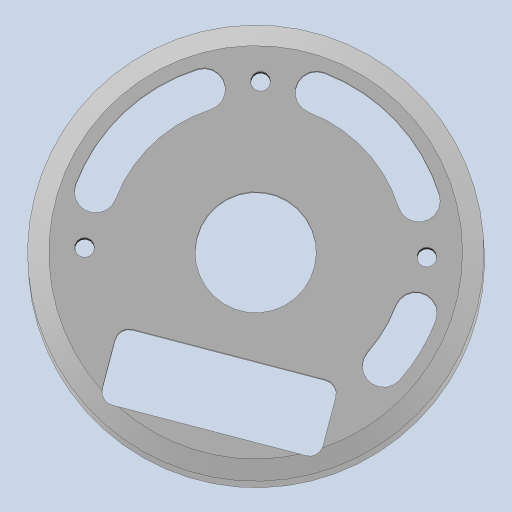
# Autodesk Inventor part: PotCover-Shorter
Saved by Autodesk Inventor 2023 (Build 270158000, 158)
## iProperties
Created: 2024-02-10
Part Number: PotCover-Shorter
Material: Generic
Document SubType Name: Modeling
Designer: LattePanda
Density: 1 g/cm^3
Appearance: Default
Author: LattePanda
Autodesk Inventor part; units mm, degrees
ref_plane "YZ Plane" through (0, 0, 0) normal (1, 0, 0) x (0, 1, 0)
ref_plane "XZ Plane" through (0, 0, 0) normal (0, 1, 0) x (-1, 0, 0)
sketch "Sketch1" plane through (0, 0, 0) normal (0, 0, 1) x (1, 0, 0)
  circle A0 centre (0, 0) radius 16
  dimension "d0" = 32
  constraints: 1 centre point, 1 coincident
  measures "d0" diameter of A0
extrude "Extrusion1" add sketch "Sketch1" along normal blind 13
sketch "Sketch2" plane through (0, 0, 0) normal (0, 0, -1) x (-1, 0, 0)
  circle A0 centre (0, 0) radius 16 projected
  circle A1 centre (0, 0) radius 14.5
  dimension "d3" = 1.5
  dimension "d11" = 29
  constraints: 1 centre point, 1 coincident
  measures "d3" radial gap between concentric circles of A0 A1
  measures "d11" diameter of A1
ref_plane "Work Plane1" through (0, 0, 11.5) normal (0, 0, 1) x (1, 0, 0)
extrude "Extrusion2" cut sketch "Sketch2" against normal up to surface (11.5 mm away) contours A1
sketch "Sketch3" plane through (0, 0, 13) normal (0, 0, 1) x (1, 0, 0)
  circle A0 centre (0, 0) radius 4.25
  dimension "d7" = 8.5
  constraints: 1 centre point, 1 coincident
  measures "d7" diameter of A0
extrude "Extrusion3" cut sketch "Sketch3" against normal through all
sketch "Sketch4" plane through (0, 0, 13) normal (0, 0, 1) x (1, 0, 0)
  circle A0 centre (0, 0) radius 4.25 construction
  circle A1 centre (0, 0) radius 16 construction
  line L0 (0, 0) -> (0, 16) construction
  circle A2 centre (0, 0) radius 16 projected
  line L1 (0, 0) -> (-16, 0) construction
  circle A3 centre (-12, 0) radius 0.7
  circle A4 centre (0, 12) radius 0.7
  circle A5 centre (12, 0) radius 0.7
  dimension "d10" = 12
  dimension "d12" = 12
  dimension "d13" = 1.4
  constraints: 4 end point, 3 centre point, 2 point on circle, 2 point on line, 1 equal radius, 1 horizontal, 1 symmetric about line, 1 vertical, 1 other
  measures "d10" distance of point (0, 0) A3.centre
  measures "d12" distance of point (0, 0) A4.centre
  measures "d13" diameter of A4
extrude "Extrusion4" cut sketch "Sketch4" against normal through all contours A3 | A4 | A5
sketch "Sketch5" plane through (0, 0, 13) normal (0, 0, 1) x (1, 0, 0)
  circle A0 centre (0, 0) radius 14.5 projected
  line L0 (-10.0993, -10.4045) -> (4.5162, -13.7787)
  line L1 (0, 0) -> (-2.7916, -12.0916) construction
  circle A1 centre (-12, 0) radius 0.7 construction
  line L2 (0, 0) -> (-12, 0) construction
  line L3 (-10.0993, -10.4045) -> (-9.0871, -6.0198)
  line L4 (-9.0871, -6.0198) -> (5.5285, -9.3941)
  line L5 (4.5162, -13.7787) -> (5.5285, -9.3941)
  dimension "d17" = 77
  dimension "d18" = 4.5
  dimension "d19" = 15
  constraints: 12 end point, 3 perpendicular, 2 point on circle, 1 horizontal, 1 midpoint
  measures "d17" angle of L2 L1
  measures "d18" distance of L0.start L3.end
  measures "d19" distance of L0.start L0.end
extrude "Extrusion5" cut sketch "Sketch5" against normal through all contours L3 L4 L5 L0
fillet "Fillet1" radius 0.5 4 edges at (-9.0871, -6.0198, 12.25) (5.5285, -9.3941, 12.25) (-10.0993, -10.4045, 12.25) (4.5162, -13.7787, 12.25)
sketch "Sketch6" plane through (0, 0, 13) normal (0, 0, 1) x (1, 0, 0)
  circle A0 centre (0, 0) radius 16 projected
  line L0 (-3.0691, 15.7029) -> (-2.234, 9.7613) construction
  line L1 (-2.234, 9.7613) -> (-4.2426, 4.2426) construction
  line L2 (0, 0) -> (-11.3137, 11.3137) construction
  circle A1 centre (0, 12) radius 0.7 construction
  line L3 (0, 0) -> (0, 12) construction
  line L4 (-15.7029, 3.0691) -> (-9.7613, 2.234) construction
  line L5 (-9.7613, 2.234) -> (-4.2426, 4.2426) construction
  line L6 (3.0691, 15.7029) -> (2.234, 9.7613) construction
  line L7 (2.234, 9.7613) -> (4.2426, 4.2426) construction
  line L8 (9.7613, 2.234) -> (4.2426, 4.2426) construction
  line L9 (15.7029, 3.0691) -> (9.7613, 2.234) construction
  line L10 (-15.5637, 4.0593) -> (-9.869, 3.259)
  line L11 (-9.869, 3.259) -> (-5.0228, 5.0228)
  line L12 (-5.0228, 5.0228) -> (-3.259, 9.869)
  line L13 (-3.259, 9.869) -> (-4.0593, 15.5637)
  line L14 (4.0593, 15.5637) -> (3.259, 9.869)
  line L15 (3.259, 9.869) -> (5.0228, 5.0228)
  line L16 (5.0228, 5.0228) -> (9.869, 3.259)
  line L17 (9.869, 3.259) -> (15.5637, 4.0593)
  point P0 (-4.0475, 15.4796)
  point P1 (-15.4796, 4.0475)
  point P2 (15.4796, 4.0475)
  point P3 (4.0475, 15.4796)
  dimension "d23" = 45
  dimension "d24" = 6
  dimension "d25" = 8
  dimension "d26" = 20
  dimension "d27" = 6
  dimension "d36" = 1
  dimension "d37" = 1
  constraints: 36 end point, 7 symmetric about line, 2 point on circle, 1 point on line, 1 vertical, 6 other
  measures "d23" angle of L3 L2
  measures "d24" distance of L0.start L0.end
  measures "d25" angle of L3 L0
  measures "d26" angle of L3 L1
  measures "d27" distance of point (0, 0) L1.end
  measures "d36" distance between parallel lines of L4 L10
  measures "d37" distance between parallel lines of L6 L14
extrude "Extrusion6" [suppressed]
chamfer "Chamfer1" distance 1.5 angle 45 1 edges at (-16, 0, 13)
sketch "Sketch8" plane through (0, 0, 13) normal (0, 0, 1) x (1, 0, 0)
  line L0 (-8.5999, -6.1323) -> (5.0413, -9.2816) construction
  arc A0 (-8.5999, -6.1323) -> (-9.1995, -6.507) centre (-8.7124, -6.6195) ccw construction
  line L1 (-9.9869, -9.9173) -> (-9.1995, -6.507) construction
  arc A1 (-9.9869, -9.9173) -> (-9.6122, -10.517) centre (-9.4997, -10.0298) ccw construction
  line L2 (4.029, -13.6663) -> (-9.6122, -10.517) construction
  arc A2 (4.029, -13.6663) -> (4.6287, -13.2916) centre (4.1415, -13.1791) ccw construction
  line L3 (5.416, -9.8813) -> (4.6287, -13.2916) construction
  arc A3 (5.416, -9.8813) -> (5.0413, -9.2816) centre (4.9288, -9.7688) ccw construction
  line L4 (5.1538, -8.7944) -> (-8.4874, -5.6451)
  arc A4 (-8.4874, -5.6451) -> (-9.6867, -6.3945) centre (-8.7124, -6.6195) ccw
  line L5 (-9.6867, -6.3945) -> (-10.4741, -9.8048)
  arc A5 (-10.4741, -9.8048) -> (-9.7246, -11.0041) centre (-9.4997, -10.0298) ccw
  line L6 (-9.7246, -11.0041) -> (3.9165, -14.1535)
  arc A6 (3.9165, -14.1535) -> (5.1159, -13.404) centre (4.1415, -13.1791) ccw
  line L7 (5.1159, -13.404) -> (5.9032, -9.9937)
  arc A7 (5.9032, -9.9937) -> (5.1538, -8.7944) centre (4.9288, -9.7688) ccw
  point P0 (0, 0)
  dimension "d38" = 0.5
  constraints: 8 end point, 8 point on circle, 4 centre point, 7 other
  measures "d38" distance between parallel lines of L0 L4
extrude "Extrusion7" cut sketch "Sketch8" against normal through all
sketch "Sketch10" plane through (0, 0, 13) normal (0, 0, 1) x (1, 0, 0)
  arc A0 (-3.9441, 11.3333) -> (-11.3333, 3.9441) centre (0, 0) ccw construction
  arc A1 (-4.4371, 12.75) -> (-12.75, 4.4371) centre (0, 0) ccw
  arc A2 (-3.451, 9.9167) -> (-9.9167, 3.451) centre (0, 0) ccw
  arc A3 (-3.451, 9.9167) -> (-4.4371, 12.75) centre (-3.9441, 11.3333) ccw
  arc A4 (-12.75, 4.4371) -> (-9.9167, 3.451) centre (-11.3333, 3.9441) ccw
  arc A5 (11.3333, 3.9441) -> (3.9441, 11.3333) centre (0, 0) ccw construction
  arc A6 (12.75, 4.4371) -> (4.4371, 12.75) centre (0, 0) ccw
  arc A7 (9.9167, 3.451) -> (3.451, 9.9167) centre (0, 0) ccw
  arc A8 (9.9167, 3.451) -> (12.75, 4.4371) centre (11.3333, 3.9441) ccw
  arc A9 (4.4371, 12.75) -> (3.451, 9.9167) centre (3.9441, 11.3333) ccw
  arc A10 (9.1909, -7.7154) -> (11.3333, -3.9441) centre (0, 0) ccw construction
  arc A11 (10.3398, -8.6798) -> (12.75, -4.4371) centre (0, 0) ccw
  arc A12 (8.042, -6.751) -> (9.9167, -3.451) centre (0, 0) ccw
  arc A13 (8.042, -6.751) -> (10.3398, -8.6798) centre (9.1909, -7.7154) ccw
  arc A14 (12.75, -4.4371) -> (9.9167, -3.451) centre (11.3333, -3.9441) ccw
  circle A15 centre (0, 0) radius 12 construction
  circle A16 centre (0, 12) radius 0.7 projected
  circle A17 centre (12, 0) radius 0.7 projected
  circle A18 centre (-12, 0) radius 0.7 projected
  point P0 (5.9032, -9.9937)
  dimension "d44" = 24
  dimension "d45" = 1.5
  dimension "d46" = 4
  dimension "d47" = 4
  dimension "d48" = 4
  dimension "d49" = 4
  dimension "d50" = 4
  dimension "d51" = 4
  constraints: 34 point on circle, 16 centre point, 12 tangent, 3 concentric, 2 equal radius, 1 coincident
  measures "d44" diameter of A15
  measures "d45" radius of A4
  measures "d46" distance of A16.centre A0.start
  measures "d47" distance of A18.centre A0.end
  measures "d48" distance of A5.start A17.centre
  measures "d49" distance of A17.centre A10.end
  measures "d50" distance of A10.start point (5.903, -9.994)
  measures "d51" distance of A16.centre A5.end
extrude "Extrusion9" cut sketch "Sketch10" against normal through all contours A3 A2 A4 A1 | A8 A7 A9 A6 | A13 A12 A14 A11
sketch "Sketch11" plane through (0, 0, 11.5) normal (0, 0, -1) x (-0.9744, 0.225, 0)
  circle A0 centre (2.6994, 11.6924) radius 0.7 projected
  circle A1 centre (11.6924, -2.6994) radius 0.7 projected
  circle A2 centre (-11.6924, 2.6994) radius 0.7 projected
  circle A3 centre (2.6994, 11.6924) radius 1.5
  circle A4 centre (-11.6924, 2.6994) radius 1.5
  circle A5 centre (11.6924, -2.6994) radius 1.5
  point P0 (0, 0)
  dimension "d54" = 3
  dimension "d55" = 3
  dimension "d56" = 3
  constraints: 3 centre point, 3 coincident
  measures "d54" diameter of A3
  measures "d55" diameter of A4
  measures "d56" diameter of A5
extrude "Extrusion10" add sketch "Sketch11" along normal blind 1.5
equation "\"d12\" = d10"
equation "\"d47\" = d46"
equation "\"d48\" = d46"
equation "\"d49\" = d46"
equation "\"d50\" = d46"
equation "\"d51\" = d46"
body "Solid1"
